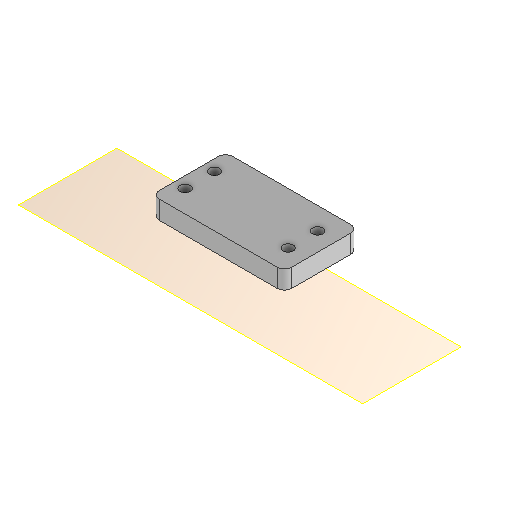
# Autodesk Inventor part: 60_Planktoscope_Cabletie
Saved by Autodesk Inventor 2024.1 (Build 281209000, 209)
## iProperties
Created: 2024-08-07
Part Number: 60_Planktoscope_Cabletie
Material: Generisch
Document SubType Name: Modeling
Designer: diederichbenedict
Density: 1 g/cm^3
Appearance: Vorgabe
Vendor: openUC2
Mass: 3.45968 g
Surface Area: 21.0263 cm^2
Volume: 3.45968 cm^3
Author: diederichbenedict
Autodesk Inventor part; units mm, degrees
ref_plane "YZ Plane" through (0, 0, 0) normal (1, 0, 0) x (0, 1, 0)
ref_plane "XZ Plane" through (0, 0, 0) normal (0, 1, 0) x (-1, 0, 0)
ref_plane "XY Plane" through (0, 0, 0) normal (0, 0, 1) x (1, 0, 0)
ref_plane "Arbeitsebene1" through (0, 0, 0) normal (0, 0, 1) x (1, 0, 0)
sketch "Skizze1" plane through (0, 0, 0) normal (0, 0, 1) x (1, 0, 0)
  circle A0 centre (86.3298, 4) radius 1.4 projected
  circle A1 centre (24.4799, 20.3) radius 1.4 projected
  circle A2 centre (52.4799, 20.3) radius 1.4 projected
  circle A3 centre (52.4799, 6.2) radius 1.4 projected
  circle A4 centre (24.4799, 6.2) radius 1.4 projected
  circle A5 centre (7.3298, 20.3) radius 1.4 projected
  circle A6 centre (7.3298, 4) radius 1.4 projected
  line L0 (90, 24.3) -> (90, 0) projected
  line L1 (89.0152, 24.3) -> (90, 24.3) projected
  line L2 (89.0152, 24.3) -> (89.0152, 10) projected
  line L3 (89.0152, 10) -> (59.35, 10) projected
  line L4 (59.35, 10) -> (59.35, 24.3) projected
  line L5 (5, 24.3) -> (59.35, 24.3) projected
  line L6 (5, 0) -> (5, 24.3) projected
  line L7 (5, 0) -> (90, 0) projected
  line L8 (6, 48.6) -> (6, 24.3) projected
  line L9 (6, 24.3) -> (60.35, 24.3) projected
  line L10 (60.35, 38.6) -> (60.35, 24.3) projected
  line L11 (89.95, 38.6) -> (60.35, 38.6) projected
  line L12 (89.95, 24.3) -> (89.95, 38.6) projected
  line L13 (89.95, 24.3) -> (91, 24.3) projected
  line L14 (91, 24.3) -> (91, 48.6) projected
  line L15 (6, 48.6) -> (91, 48.6) projected
  line L16 (21.4799, 24.3) -> (57.4799, 24.3)
  line L17 (57.4799, 24.3) -> (57.4799, 14.3)
  line L18 (57.4799, 14.3) -> (21.4799, 14.3)
  line L19 (21.4799, 14.3) -> (21.4799, 24.3)
  point P0 (0, 0)
  dimension "d0" = 36
  dimension "d1" = 10
  dimension "d2" = 3
  constraints: 8 end point, 2 parallel, 1 horizontal, 1 perpendicular, 1 point on line
  measures "d0" distance of L17.end L18.end
  measures "d1" distance of L16.end L17.end
  measures "d2" distance from line of L19 A1.centre
extrude "Extrusion1" add sketch "Skizze1" along normal blind 5 contours L5 L17 L18 L19
fillet "Rundung1" radius 2 2 edges at (21.4799, 14.3, 2.5) (57.4799, 14.3, 2.5)
mirror "Spiegeln1" about plane through (57.4799, 24.3, 0) normal (0, 1, 0) of "Extrusion1", "Rundung1"
